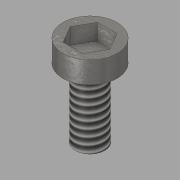
# Autodesk Inventor part: Electronics Mounting bolt
Saved by Autodesk Inventor 2017 (Build 210142000, 142)
## iProperties
Created: 2017-01-17
Part Number: Electronics Mounting bolt
Material: Steel, Galvanized
Document SubType Name: Modeling
Designer: qupec
Density: 7.85 g/cm^3
Appearance: Galvanized
Author: qupec
Autodesk Inventor part; units mm, degrees
ref_plane "YZ Plane" through (0, 0, 0) normal (1, 0, 0) x (0, 1, 0)
ref_plane "XZ Plane" through (0, 0, 0) normal (0, 1, 0) x (-1, 0, 0)
ref_plane "XY Plane" through (0, 0, 0) normal (0, 0, 1) x (1, 0, 0)
sketch "Sketch1" plane through (0, 0, 0) normal (0, 1, 0) x (-1, 0, 0)
  circle A0 centre (0, 0) radius 1.365
  dimension "d0" = 2.73
  constraints: 1 centre point, 1 coincident
  measures "d0" diameter of A0
extrude "Extrusion1" add sketch "Sketch1" along normal blind 6.35
sketch "Sketch2" plane through (0, 6.35, 0) normal (0, 1, 0) x (1, 0, 0)
  circle A0 centre (0, 0) radius 2.5
  dimension "d3" = 5
  constraints: 1 centre point, 1 coincident
  measures "d3" diameter of A0
extrude "Extrusion2" add sketch "Sketch2" along normal blind 2
sketch "Sketch3" plane through (0, 8.35, 0) normal (0, 1, 0) x (1, 0, 0)
  circle A0 centre (0, 0) radius 1.365 projected
  line L0 (-1.8331, 0) -> (-0.9165, 1.5875)
  line L1 (-0.9165, 1.5875) -> (0.9165, 1.5875)
  line L2 (0.9165, 1.5875) -> (1.8331, 0)
  line L3 (1.8331, 0) -> (0.9165, -1.5875)
  line L4 (0.9165, -1.5875) -> (-0.9165, -1.5875)
  line L5 (-0.9165, -1.5875) -> (-1.8331, 0)
  dimension "d6" = 3.175
  constraints: 12 end point, 1 coincident, 13 other
  measures "d6" distance between parallel lines of L1 L4
extrude "Extrusion3" cut sketch "Sketch3" against normal blind 1.5 contours A0 | L0 L1 L2 L3 L4 L5
thread "Thread1" size "4-40 UNC" class "2A" standard "ANSI Unified Screw Threads" full length
body "Solid1"
